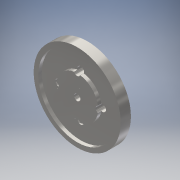
# Autodesk Inventor part: Shaft
Saved by Autodesk Inventor 2016 (Build 200138000, 138)
## iProperties
Created: 2017-12-07
Part Number: Shaft
Material: Generic
Document SubType Name: Modeling
Designer: student
Density: 1 g/cm^3
Appearance: Default
Author: student
Autodesk Inventor part; units mm, degrees
ref_plane "YZ Plane" through (0, 0, 0) normal (1, 0, 0) x (0, 1, 0)
ref_plane "XY Plane" through (0, 0, 0) normal (0, 0, 1) x (1, 0, 0)
sketch "Sketch1" plane through (0, 0, 0) normal (0, 0, 1) x (1, 0, 0)
  circle A0 centre (0, 0) radius 21.59
  dimension "d0" = 43.18
  constraints: 1 centre point, 1 coincident
  measures "d0" diameter of A0
extrude "Extrusion1" add sketch "Sketch1" along normal blind 5.08
sketch "Sketch2" plane through (0, 0, 5.08) normal (0, 0, 1) x (1, 0, 0)
  circle A0 centre (0, 0) radius 10.3632
  circle A1 centre (0, 0) radius 19.304
  dimension "d3" = 20.7264
  dimension "d4" = 38.608
  constraints: 2 centre point, 2 coincident
  measures "d3" diameter of A0
  measures "d4" diameter of A1
extrude "Extrusion2" cut sketch "Sketch2" against normal blind 1.7272
sketch "Sketch3" plane through (0, 0, 5.08) normal (0, 0, 1) x (1, 0, 0)
  circle A0 centre (0, 0) radius 4.572
  dimension "d7" = 9.144
  constraints: 1 centre point, 1 coincident
  measures "d7" diameter of A0
extrude "Extrusion3" add sketch "Sketch3" along normal blind 0.0025 and the other way blind 12.7
sketch "Sketch5" plane through (0, 0, 5.0825) normal (0, 0, 1) x (1, 0, 0)
  arc A0 (-1.2065, -1.0318) -> (-1.2065, 1.0318) centre (0, 0) ccw
  line L0 (-1.2065, -1.0318) -> (-1.2065, 1.0318)
  constraints: 2 end point, 2 point on circle, 1 centre point, 1 coincident, 1 vertical
extrude "Extrusion5" cut sketch "Sketch5" against normal blind 11.43
sketch "Sketch6" plane through (0, 0, 5.0825) normal (0, 0, 1) x (1, 0, 0)
  circle A0 centre (0, 0) radius 1.5875
  dimension "d19" = 3.175
  constraints: 1 centre point, 1 coincident
  measures "d19" diameter of A0
extrude "Extrusion6" cut sketch "Sketch6" against normal blind 4.572
sketch "Sketch8" plane through (0, 0, 0) normal (0, 0, -1) x (-1, 0, 0)
  circle A0 centre (0, 0) radius 10.3632 projected
  circle A1 centre (10.8585, 0) radius 1.6891
  circle A2 centre (-10.8585, 0) radius 1.6891
  circle A3 centre (0, 0) radius 4.572 projected
  circle A4 centre (0, 0) radius 6.6294 projected
  circle A5 centre (0, -10.8585) radius 1.6891
  circle A6 centre (0, 10.8585) radius 1.6891
  dimension "d25" = 3.3782
  dimension "d26" = 3.3782
  dimension "d29" = 3.3782
  dimension "d30" = 3.3782
  dimension "d38" = 10.8585
  dimension "d39" = 10.8585
  dimension "d40" = 10.8585
  dimension "d41" = 10.8585
  constraints: 4 centre point
  measures "d25" diameter of A1
  measures "d26" diameter of A2
  measures "d29" diameter of A5
  measures "d30" diameter of A6
  measures "d38" distance of A4.centre A2.centre
  measures "d39" distance of A4.centre A1.centre
  measures "d40" distance of A4.centre A6.centre
  measures "d41" distance of A4.centre A5.centre
extrude "Extrusion8" cut sketch "Sketch8" against normal blind 25.4 contours A0 A1 | A0 A1 | A6 A0 | A0 A6 | A5 A0 | A0 A5 | A2 A0 | A0 A2
ref_plane "Work Plane1" through (0, 4.572, 5.08) normal (0, 1, 0) x (-1, 0, 0)
sketch "Sketch9" plane through (0, 4.572, 5.08) normal (0, 1, 0) x (-1, 0, 0)
  circle A0 centre (0, -9.7924) radius 1.27
  point P0 (0, -5.08)
  dimension "d35" = 2.54
  constraints: 1 centre point
  measures "d35" diameter of A0
extrude "Extrusion9" cut sketch "Sketch9" against normal blind 25.4
body "Solid1"
